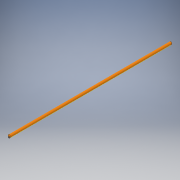
# Autodesk Inventor part: cables
Saved by Autodesk Inventor 2017 (Build 210142000, 142)
## iProperties
Created: 2018-12-03
Part Number: cables
Material: Generic
Document SubType Name: Modeling
Designer: ddeboer
Density: 1 g/cm^3
Appearance: Default
Author: ddeboer
Autodesk Inventor part; units mm, degrees
ref_plane "YZ Plane" through (0, 0, 0) normal (1, 0, 0) x (0, 1, 0)
ref_plane "XZ Plane" through (0, 0, 0) normal (0, 1, 0) x (-1, 0, 0)
ref_plane "XY Plane" through (0, 0, 0) normal (0, 0, 1) x (1, 0, 0)
sketch "Sketch1" plane through (0, 0, 0) normal (0, 0, 1) x (1, 0, 0)
  circle A0 centre (6.7942, 9.4603) radius 5
  circle A1 centre (4.6245, 2.6147) radius 2
  circle A2 centre (7.612, 3.4573) radius 1
  circle A3 centre (2.4796, 4.9893) radius 1
  point P0 (0, 0)
  dimension "d0" = 10
  dimension "d1" = 4
  dimension "d2" = 2
  dimension "d3" = 2
  constraints: 4 centre point
  measures "d0" diameter of A0
  measures "d1" diameter of A1
  measures "d2" diameter of A2
  measures "d3" diameter of A3
extrude "Extrusion1" add sketch "Sketch1" along normal blind 650
sketch "Sketch2" plane through (6.7942, 9.4603, 650) normal (0, 0, 1) x (1, 0, 0)
  line L0 (-2.1527, -6.9412) -> (0.9548, 3.0788) construction
  circle A0 centre (-0.5989, -1.9312) radius 0.8997
  constraints: 2 end point, 1 centre point, 1 midpoint
hole "Hole1" at (6.1953, 7.5291, 650) direction (0, 0, -1) diameter 1.8 depth 2 tip angle 118
body "Solid1"
